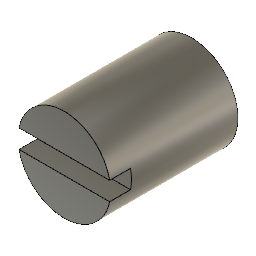
_m8 nut.b4a01997-4159-4649-9a80-1123b2736154 (Autodesk Fusion 360 design; units mm, degrees)
Autodesk Fusion 360 part; units mm, degrees
sketch "Sketch1" plane through (0, 0, 0) normal (0, 1, 0) x (1, 0, 0)
  circle A0 centre (0, 0) radius 4
  dimension "d1" = 8
  constraint coincident A0.centre origin
  measures "d1" diameter of A0
extrude "Extrude1" add sketch "Sketch1" along normal blind 11
sketch "Sketch2" plane through (0, 0, 0) normal (1, 0, 0) x (0, 1, 0)
  line L0 (0, -4) -> (0, 4)
  line L1 (0, 0) -> (0, 0.8)
  line L2 (0, 0.8) -> (0, -0.8)
  line L3 (0, 0) -> (0, 0.8)
  line L4 (0, 0.8) -> (0, -0.8)
  line L5 (0, 0.8) -> (1.8, 0.8)
  line L6 (1.8, 0.8) -> (1.8, -0.8)
  line L7 (1.8, -0.8) -> (0, -0.8)
  dimension "d6" = 0.8
  dimension "d7" = 1.6
  dimension "d8" = 1.8
  dimension "d9" = 1.6
  constraint coincident L1.start L3.start
  constraint parallel L0 L1
  constraint parallel L0 L2
  constraint parallel L1 L3
  constraint parallel L2 L4
  constraint perpendicular L0 L5
  constraint perpendicular L5 L6
  constraint perpendicular L0 L7
  measures "d6" distance of L1.start L1.end
  measures "d7" distance of L1.end L2.end
  measures "d8" distance of L1.end L5.end
  measures "d9" distance of L5.end L6.end
extrude "Extrude2" cut sketch "Sketch2" along normal blind 5.3 and the other way blind 4.5
